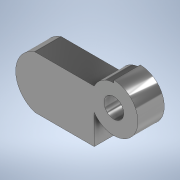
# Autodesk Inventor part: Parte98
Saved by Autodesk Inventor 2021 (Build 250183000, 183)
## iProperties
Created: 2020-12-03
Part Number: Parte98
Material: Liga de Nickel-Copper 400
Document SubType Name: Modeling
Designer: Lucas Moura
Density: 8.83 g/cm^3
Appearance: Cromado - Preto polido
Author: Lucas Moura
Autodesk Inventor part; units mm, degrees
ref_plane "YZ Plane" through (0, 0, 0) normal (1, 0, 0) x (0, 1, 0)
ref_plane "XZ Plane" through (0, 0, 0) normal (0, 1, 0) x (-1, 0, 0)
ref_plane "XY Plane" through (0, 0, 0) normal (0, 0, 1) x (1, 0, 0)
sketch "Sketch1" plane through (0, 0, 0) normal (0, 0, 1) x (1, 0, 0)
  circle A0 centre (5.0032, 3.2866) radius 1.82
  point P0 (0, 0)
  dimension "d0" = 3.64
  constraints: 1 centre point
  measures "d0" diameter of A0
extrude "Extrusion1" add sketch "Sketch1" along normal blind 2
sketch "Sketch2" plane through (5.0032, 3.2866, 2) normal (0, 0, 1) x (1, 0, 0)
  circle A0 centre (0, 0) radius 0.75
  point P0 (-5.0032, -3.2866)
  dimension "d3" = 1.5
  constraints: 1 centre point
  measures "d3" diameter of A0
extrude "Extrusion2" cut sketch "Sketch2" against normal through all
sketch "Sketch3" plane through (5.0032, 3.2866, 2) normal (0, 0, 1) x (1, 0, 0)
  line L0 (0, -1.82) -> (0, -0.682) construction
  line L1 (-1.6874, -0.682) -> (-1.4874, -0.682)
  circle A0 centre (0, 0) radius 1.82 projected
  circle A1 centre (0, 0) radius 1.6363
  line L2 (0, 1.6363) -> (0, 1.82)
  point P0 (-5.0032, -3.2866)
  point P1 (0.02, 0)
  dimension "d6" = 1.138
  dimension "d7" = 0.2
  constraints: 6 end point, 3 point on circle, 2 vertical, 1 centre point, 1 coincident
  measures "d6" distance of L0.start L0.end
  measures "d7" distance of L1.start L1.end
extrude "Extrusion3" cut sketch "Sketch3" against normal through all contours A0 L2 A1 L1 picked at (-0.267, 1.7273)
sketch "Sketch5" plane through (0, 0, 0) normal (0, 0, -1) x (-1, 0, 0)
  line L0 (-3.3158, 2.6046) -> (-3.5158, 2.6046) projected
  arc A0 (-3.5158, 2.6046) -> (-5.0032, 4.9229) centre (-5.0032, 3.2866) ccw projected
  line L1 (-5.0032, 4.9229) -> (-5.0032, 5.1066) projected
  arc A1 (-5.0032, 5.1066) -> (-3.3158, 2.6046) centre (-5.0032, 3.2866) ccw projected
  circle A2 centre (-5.0032, 3.2866) radius 0.75 projected
  line L2 (-3.5158, 2.6046) -> (-3.5158, 2.2377) construction
  arc A3 (-5.0032, 5.1066) -> (-3.3158, 2.6046) centre (-5.0032, 3.2866) ccw projected
  line L3 (-3.5158, 3.9686) -> (-3.5158, 0)
  line L4 (-3.5158, 0) -> (0.9842, 0)
  line L5 (0.9842, 0) -> (0.9842, 3.9686)
  line L6 (0.9842, 3.9686) -> (-3.5158, 3.9686)
  arc A4 (0.9842, 0) -> (0.9842, 3.9686) centre (0.3524, 1.9843) ccw
  point P0 (0, 0)
  dimension "d18" = 4.5
  constraints: 10 end point, 4 point on circle, 3 perpendicular, 2 point on line, 1 centre point, 1 vertical
  measures "d18" distance of L5.end L3.start
extrude "Extrusion6" add sketch "Sketch5" against normal up to surface (2 mm away) contours L0 A0 L6 L5 L4 L3 A1 | A4 L5
body "Solid1"
